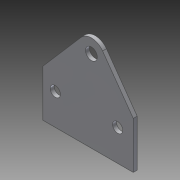
# Autodesk Inventor part: Bracket
Saved by Autodesk Inventor 2014 SP1 (Build 180222100, 222)
## iProperties
Created: 2014-01-06
Part Number: Bracket
Material: Aluminum 6061
Document SubType Name: Modeling
Designer: Andrew Toennies
Density: 2.71 g/cm^3
Appearance: Aluminum - Flat
Mass: 4.62013 g
Surface Area: 24.2033 cm^2
Volume: 1.70484 cm^3
Author: Andrew Toennies
Autodesk Inventor part; units mm, degrees
ref_plane "YZ Plane" through (0, 0, 0) normal (1, 0, 0) x (0, 1, 0)
ref_plane "XZ Plane" through (0, 0, 0) normal (0, 1, 0) x (-1, 0, 0)
ref_plane "XY Plane" through (0, 0, 0) normal (0, 0, 1) x (1, 0, 0)
sketch "Sketch1" plane through (0, 0, 0) normal (0, 0, 1) x (1, 0, 0)
  circle A0 centre (0, 0) radius 2.0828
  circle A1 centre (25.4, 0) radius 2.0828
  line L0 (25.4, 0) -> (0, 0) construction
  line L1 (-5.08, 6.35) -> (31.75, 6.35) construction
  line L2 (31.75, 6.35) -> (31.75, -12.7)
  line L3 (31.75, -12.7) -> (-5.08, -12.7)
  line L4 (-5.08, -12.7) -> (-5.08, 6.35)
  circle A2 centre (14.7013, 20.6375) radius 2.413 projected
  arc A3 (19.2514, 23.8814) -> (10.479, 24.2978) centre (14.7013, 20.6375) ccw
  line L5 (-5.08, 6.35) -> (10.479, 24.2978)
  line L6 (31.75, 6.35) -> (19.2514, 23.8814)
  dimension "d0" = 4.1656
  dimension "d1" = 4.1656
  dimension "d5" = 12.7
  dimension "d6" = 6.35
  dimension "d7" = 5.08
  dimension "d8" = 11.176
  dimension "d9" = 6.35
  dimension "d10" = 25.4
  constraints: 14 end point, 3 centre point, 2 coincident, 2 horizontal, 2 parallel, 2 point on circle, 2 tangent, 1 perpendicular
  measures "d0" diameter of A0
  measures "d1" diameter of A1
  measures "d5" distance from line of L3 L0.start
  measures "d6" distance from line of L2 L0.start
  measures "d7" distance from line of L4 point (0, 0)
  measures "d8" diameter of A3
  measures "d9" distance from line of L1 L0.start
  measures "d10" distance of point (0, 0) L0.start
extrude "Extrusion1" add sketch "Sketch1" along normal blind 1.5875 contours L2 L3 L4 L5 A3 L6 | A2
sketch "Sketch2" plane through (0, 0, 0) normal (0, 0, -1) x (-1, 0, 0)
  arc A0 (-10.479, 24.2978) -> (-19.2514, 23.8814) centre (-14.7013, 20.6375) ccw projected
  circle A1 centre (-14.7013, 20.6375) radius 2.413
  dimension "d11" = 4.826
  constraints: 1 centre point, 1 coincident
  measures "d11" diameter of A1
extrude "Extrusion2" cut sketch "Sketch2" against normal blind 25.4
body "Solid1"
